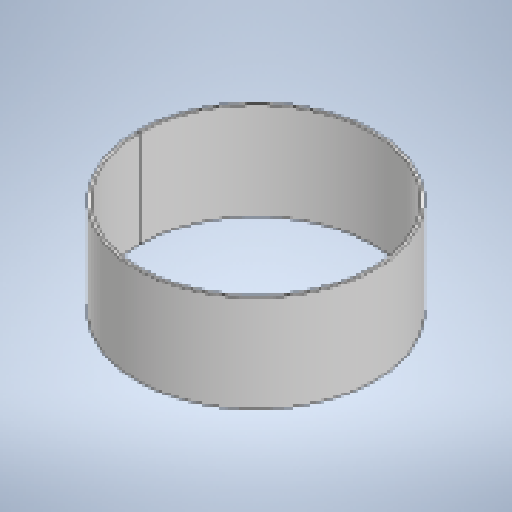
# Autodesk Inventor part: PNS-611 accses hatch tube
Saved by Autodesk Inventor 2025 (Build 290162010, 162A)
## iProperties
Created: 2025-02-12
Part Number: PNS-611 accses hatch tube
Material: Generic
Document SubType Name: Sheet Metal
Designer: pokla
Density: 1 g/cm^3
Flat Pattern Width: 168.116 cm
Flat Pattern Length: 22 cm
Flat Pattern Area: 3698.56 cm^2
Sheet Metal Rule: Default_mm
Sheet Metal Width: 1681,165 mm
Sheet Metal Length: 220,000 mm
Sheet Metal Area: 369856,211 mm^2
Appearance: Default
Mass: 1619.32 g
Surface Area: 5634.28 cm^2
Volume: 1619.32 cm^3
Author: pokla
Autodesk Inventor part; units mm, degrees
ref_plane "YZ Plane" through (0, 0, 0) normal (1, 0, 0) x (0, 1, 0)
ref_plane "XZ Plane" through (0, 0, 0) normal (0, 1, 0) x (-1, 0, 0)
ref_plane "XY Plane" through (0, 0, 0) normal (0, 0, 1) x (1, 0, 0)
sketch "Sketch1" plane through (0, 0, 0) normal (0, 1, 0) x (-1, 0, 0)
  line L0 (265, 120) -> (265, 0)
  line L1 (265, 0) -> (271, 0)
  line L2 (0, 0) -> (0, 109.131)
  line L3 (265, 120) -> (271, 120)
  line L4 (271, 0) -> (271, 120)
  line L5 (271, 0) -> (265, 0)
  line L6 (265, 0) -> (265, -100)
  line L7 (265, -100) -> (271, -100)
  line L8 (271, -100) -> (271, 0)
  point P0 (268, 0)
  point P1 (271, 0)
  dimension "d3" = 6
  dimension "d4" = 530
  dimension "d5" = 120
  dimension "d7" = 6
  dimension "d8" = 100
  constraints: 18 end point, 2 horizontal, 2 midpoint, 2 parallel, 2 perpendicular, 2 vertical, 1 horizontal alignment
  measures "d3" distance of L0.end L1.end
  measures "d4" diameter of L0 L2
  measures "d5" distance between parallel lines of L1 L3
  measures "d7" distance of L6.end L7.end
  measures "d8" distance of L7.end L5.start
revolve "Revolution1" add sketch "Sketch1" angle 359.9 about axis through (0, 0, 0) along (0, 0, 1)
sketch "Sketch2" plane through (0, 0, 0) normal (0, 1, 0) x (-1, 0, 0)
  circle A0 centre (0, -476) radius 476
  point P0 (0, 0)
  dimension "d9" = 952
  constraints: 2 vertical alignment, 2 other
extrude "Extrusion1" [suppressed]
equation "\"d4\" = Accsess_hatch_diameter"
equation "\"d5\" = Accsess_hatch_lenght"
equation "\"d7\" = d3"
equation "\"BendRadius\" = Thickness"
equation "\"BendReliefWidth\" = Thickness"
equation "\"BendReliefDepth\" = 0.5 * Thickness"
equation "\"CornerReliefSize\" = 4 * Thickness"
equation "\"MinimumRemnant\" = 2 * Thickness"
equation "\"TransitionRadius\" = BendRadius"
equation "\"JacobiRadiusSize\" = BendRadius"
equation "\"GapSize\" = Thickness"
equation "\"Accsess_hatch_diameter\" = 530"
equation "\"Accsess_hatch_lenght\" = 120"
equation "\"Thickness\" = 6"
body "Solid1"
